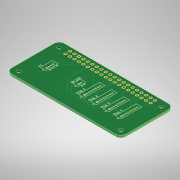
# Autodesk Inventor part: board_main
Saved by Autodesk Inventor 2022.2 (Build 262287010, 287A)
## iProperties
Created: 2025-12-30
Part Number: board_main
Material: Generic
Document SubType Name: Modeling
Designer: dbstj
Density: 1 g/cm^3
Appearance: 매끄러움 - 짙은 산림 녹색
Author: dbstj
Autodesk Inventor part; units mm, degrees
ref_plane "YZ Plane" through (0, 0, 0) normal (1, 0, 0) x (0, 1, 0)
ref_plane "XZ Plane" through (0, 0, 0) normal (0, 1, 0) x (-1, 0, 0)
ref_plane "XY Plane" through (0, 0, 0) normal (0, 0, 1) x (1, 0, 0)
sketch "스케치1" plane through (0, 0, 0) normal (0, 1, 0) x (-1, 0, 0)
  line L0 (-29.5, -15) -> (29.5, -15)
  line L1 (32.5, -12) -> (32.5, 12)
  line L2 (29.5, 15) -> (-29.5, 15)
  line L3 (-32.5, 12) -> (-32.5, -12)
  line L4 (-32.5, -15) -> (32.5, 15) construction
  line L5 (32.5, -15) -> (-32.5, 15) construction
  line L6 (-29, -11.5) -> (29, -11.5)
  line L7 (29, -11.5) -> (29, 11.5)
  line L8 (29, 11.5) -> (-29, 11.5)
  line L9 (-29, 11.5) -> (-29, -11.5)
  line L10 (-29, -11.5) -> (29, 11.5) construction
  line L11 (29, -11.5) -> (-29, 11.5) construction
  circle A0 centre (29, 11.5) radius 1.1
  circle A1 centre (29, -11.5) radius 1.1
  circle A2 centre (-29, -11.5) radius 1.1
  circle A3 centre (-29, 11.5) radius 1.1
  arc A4 (29.5, -15) -> (32.5, -12) centre (29.5, -12) ccw
  arc A5 (-32.5, -12) -> (-29.5, -15) centre (-29.5, -12) ccw
  arc A6 (-29.5, 15) -> (-32.5, 12) centre (-29.5, 12) ccw
  arc A7 (32.5, 12) -> (29.5, 15) centre (29.5, 12) ccw
  point P0 (0, 0)
  point P1 (0, 0)
  point P2 (0, 0)
  dimension "d0" = 65
  dimension "d1" = 30
  dimension "d2" = 58
  dimension "d3" = 23
  dimension "d4" = 2.2
  dimension "d5" = 2.2
  dimension "d6" = 2.2
  dimension "d7" = 2.2
  dimension "d8" = 3
  constraints: 24 end point, 8 centre point, 8 point on circle, 8 point on line, 8 tangent, 5 coincident, 5 midpoint, 4 parallel, 3 equal radius, 2 horizontal, 2 perpendicular
  measures "d0" distance of L5.end L4.end
  measures "d1" distance of L4.end L5.start
  measures "d2" distance of L8.end L7.end
  measures "d3" distance of L7.end L6.end
  measures "d4" diameter of A0
  measures "d5" diameter of A1
  measures "d6" diameter of A2
  measures "d7" diameter of A3
  measures "d8" radius of A4
extrude "돌출1" add sketch "스케치1" along normal blind 1.2 contours A5 L3 A6 L2 A7 L1 A4 L0 | A2 L9 A3 L8 A0 L7 A1 L6
sketch "스케치2" plane through (0, 1.2, 0) normal (0, 1, 0) x (1, 0, 0)
  line L0 (29.5, 15) -> (-29.5, 15) projected
  circle A0 centre (-29, 11.5) radius 1.1 projected
  point P0 (0, 0)
  point P1 (0, 0)
  point P2 (24.13, 12.77)
  point P3 (24.13, 10.23)
  point P4 (21.59, 10.23)
  point P5 (19.05, 12.77)
  point P6 (16.51, 12.77)
  point P7 (13.97, 12.77)
  point P8 (11.43, 12.77)
  point P9 (8.89, 12.77)
  point P10 (6.35, 12.77)
  point P11 (3.81, 12.77)
  point P12 (1.27, 12.77)
  point P13 (-1.27, 12.77)
  point P14 (-3.81, 12.77)
  point P15 (-6.35, 12.77)
  point P16 (-8.89, 12.77)
  point P17 (-11.43, 12.77)
  point P18 (-13.97, 12.77)
  point P19 (-16.51, 12.77)
  point P20 (-19.05, 12.77)
  point P21 (-21.59, 12.77)
  point P22 (19.05, 10.23)
  point P23 (16.51, 10.23)
  point P24 (13.97, 10.23)
  point P25 (11.43, 10.23)
  point P26 (8.89, 10.23)
  point P27 (6.35, 10.23)
  point P28 (3.81, 10.23)
  point P29 (1.27, 10.23)
  point P30 (-1.27, 10.23)
  point P31 (-3.81, 10.23)
  point P32 (-6.35, 10.23)
  point P33 (-8.89, 10.23)
  point P34 (-11.43, 10.23)
  point P35 (-13.97, 10.23)
  point P36 (-16.51, 10.23)
  point P37 (-19.05, 10.23)
  point P38 (-21.59, 10.23)
  point P39 (-24.13, 10.23)
  point P40 (-24.13, 12.77)
  point P41 (21.59, 12.77)
  dimension "d11" = 2.54
  dimension "d12" = 2.54
  dimension "d13" = 2.54
  dimension "d14" = 2.54
  dimension "d15" = 2.54
  dimension "d16" = 2.54
  dimension "d17" = 2.54
  dimension "d18" = 2.54
  dimension "d19" = 2.54
  dimension "d20" = 2.54
  dimension "d21" = 2.54
  dimension "d22" = 2.54
  dimension "d23" = 2.54
  dimension "d24" = 2.54
  dimension "d25" = 2.54
  dimension "d26" = 2.54
  dimension "d27" = 2.54
  dimension "d29" = 2.54
  dimension "d30" = 2.54
  dimension "d31" = 2.54
  dimension "d34" = 27.73
  dimension "d35" = 2.23
  constraints: 38 horizontal alignment, 20 vertical alignment
  measures "d11" distance of point (-21.59, 12.77) point (-19.05, 12.77)
  measures "d12" distance of point (-16.51, 12.77) point (-19.05, 12.77)
  measures "d13" distance of point (-13.97, 12.77) point (-16.51, 12.77)
  measures "d14" distance of point (-11.43, 12.77) point (-13.97, 12.77)
  measures "d15" distance of point (-8.89, 12.77) point (-11.43, 12.77)
  measures "d16" distance of point (-6.35, 12.77) point (-8.89, 12.77)
  measures "d17" distance of point (-3.81, 12.77) point (-6.35, 12.77)
  measures "d18" distance of point (-1.27, 12.77) point (-3.81, 12.77)
  measures "d19" distance of point (1.27, 12.77) point (-1.27, 12.77)
  measures "d20" distance of point (3.81, 12.77) point (1.27, 12.77)
  measures "d21" distance of point (6.35, 12.77) point (3.81, 12.77)
  measures "d22" distance of point (8.89, 12.77) point (6.35, 12.77)
  measures "d23" distance of point (11.43, 12.77) point (8.89, 12.77)
  measures "d24" distance of point (13.97, 12.77) point (11.43, 12.77)
  measures "d25" distance of point (16.51, 12.77) point (13.97, 12.77)
  measures "d26" distance of point (19.05, 12.77) point (16.51, 12.77)
  measures "d27" distance of point (24.13, 12.77) point (24.13, 10.23)
  measures "d29" distance of point (21.59, 12.77) point (19.05, 12.77)
  measures "d30" distance of point (24.13, 12.77) point (21.59, 12.77)
  measures "d31" distance of point (-21.59, 12.77) point (-24.13, 12.77)
  measures "d34" horizontal distance of point (-1.27, 12.77) A0.centre
  measures "d35" distance from line of point (-24.13, 12.77) L0
hole "구멍1" at (24.13, 1.2, -12.77) at (24.13, 1.2, -10.23) at (21.59, 1.2, -10.23) at (19.05, 1.2, -12.77) at (16.51, 1.2, -12.77) at (13.97, 1.2, -12.77) at (11.43, 1.2, -12.77) at (8.89, 1.2, -12.77) at (6.35, 1.2, -12.77) at (3.81, 1.2, -12.77) at (1.27, 1.2, -12.77) at (-1.27, 1.2, -12.77) at (-3.81, 1.2, -12.77) at (-6.35, 1.2, -12.77) at (-8.89, 1.2, -12.77) at (-11.43, 1.2, -12.77) at (-13.97, 1.2, -12.77) at (-16.51, 1.2, -12.77) at (-19.05, 1.2, -12.77) at (-21.59, 1.2, -12.77) at (19.05, 1.2, -10.23) at (16.51, 1.2, -10.23) at (13.97, 1.2, -10.23) at (11.43, 1.2, -10.23) at (8.89, 1.2, -10.23) at (6.35, 1.2, -10.23) at (3.81, 1.2, -10.23) at (1.27, 1.2, -10.23) at (-1.27, 1.2, -10.23) at (-3.81, 1.2, -10.23) at (-6.35, 1.2, -10.23) at (-8.89, 1.2, -10.23) at (-11.43, 1.2, -10.23) at (-13.97, 1.2, -10.23) at (-16.51, 1.2, -10.23) at (-19.05, 1.2, -10.23) at (-21.59, 1.2, -10.23) at (-24.13, 1.2, -10.23) at (-24.13, 1.2, -12.77) at (21.59, 1.2, -12.77) direction (0, -1, 0) diameter 1 end through all
sketch "스케치3" plane through (0, 1.2, 0) normal (0, 1, 0) x (1, 0, 0)
  line L0 (32.5, -12) -> (32.5, 12) projected
  line L1 (29.5, 15) -> (-29.5, 15) projected
  line L2 (-32.5, 12) -> (-32.5, -12) projected
  point P0 (0, 0)
  point P1 (22.5, 4.25)
  point P2 (22.5, 3)
  point P3 (22.5, 1.75)
  point P4 (22.5, 0.5)
  point P5 (22.5, -0.75)
  point P6 (22.5, -2)
  point P7 (22.5, -3.25)
  point P8 (22.5, -4.5)
  point P9 (15.5, -4.5)
  point P10 (15.5, -3.25)
  point P11 (15.5, -2)
  point P12 (15.5, -0.75)
  point P13 (15.5, 0.5)
  point P14 (15.5, 1.75)
  point P15 (15.5, 3)
  point P16 (15.5, 4.25)
  point P17 (8.5, -4.5)
  point P18 (8.5, -3.25)
  point P19 (8.5, -2)
  point P20 (8.5, -0.75)
  point P21 (8.5, 0.5)
  point P22 (8.5, 1.75)
  point P23 (8.5, 3)
  point P24 (8.5, 4.25)
  point P25 (1.5, -4.5)
  point P26 (1.5, -3.25)
  point P27 (1.5, -2)
  point P28 (1.5, -0.75)
  point P29 (1.5, 0.5)
  point P30 (1.5, 1.75)
  point P31 (1.5, 3)
  point P32 (1.5, 4.25)
  point P33 (-5.5, 0.5)
  point P34 (-5.5, -0.75)
  point P35 (-22.5, 1.75)
  point P36 (-22.5, 0.5)
  point P37 (-22.5, -0.75)
  point P38 (-22.5, -2)
  dimension "d43" = 1.25
  dimension "d44" = 1.25
  dimension "d45" = 1.25
  dimension "d46" = 1.25
  dimension "d47" = 1.25
  dimension "d48" = 1.25
  dimension "d49" = 1.25
  dimension "d50" = 10
  dimension "d54" = 7
  dimension "d59" = 1.25
  dimension "d60" = 1.25
  dimension "d61" = 1.25
  dimension "d62" = 1.25
  dimension "d64" = 10
  dimension "d65" = 7
  dimension "d73" = 19.5
  dimension "d74" = 15.75
  dimension "d75" = 17
  constraints: 11 vertical alignment, 2 horizontal alignment, 1 horizontal, 24 other
  measures "d43" distance of point (22.5, 3) point (22.5, 4.25)
  measures "d44" distance of point (22.5, 1.75) point (22.5, 3)
  measures "d45" distance of point (22.5, 0.5) point (22.5, 1.75)
  measures "d46" distance of point (22.5, -0.75) point (22.5, 0.5)
  measures "d47" distance of point (22.5, -0.75) point (22.5, -2)
  measures "d48" distance of point (22.5, -2) point (22.5, -3.25)
  measures "d49" distance of point (22.5, -3.25) point (22.5, -4.5)
  measures "d50" distance from line of L0 point (22.5, 4.25)
  measures "d54" distance of point (22.5, -4.5) point (15.5, -4.5)
  measures "d59" distance of point (-22.5, 0.5) point (-22.5, 1.75)
  measures "d60" distance of point (-22.5, -0.75) point (-22.5, 0.5)
  measures "d61" distance of point (-22.5, -2) point (-22.5, -0.75)
  measures "d62" distance of point (-5.5, -0.75) point (-5.5, 0.5)
  measures "d64" distance from line of L2 point (-22.5, 1.75)
  measures "d65" horizontal distance of point (1.5, 4.25) point (-5.5, 0.5)
  measures "d73" distance from line of L1 point (22.5, -4.5)
  measures "d74" distance from line of L1 point (-5.5, -0.75)
  measures "d75" distance from line of L1 point (-22.5, -2)
hole "구멍2" at (22.5, 1.2, -4.25) at (22.5, 1.2, -3) at (22.5, 1.2, -1.75) at (22.5, 1.2, -0.5) at (22.5, 1.2, 0.75) at (22.5, 1.2, 2) at (22.5, 1.2, 3.25) at (22.5, 1.2, 4.5) at (15.5, 1.2, 4.5) at (15.5, 1.2, 3.25) at (15.5, 1.2, 2) at (15.5, 1.2, 0.75) at (15.5, 1.2, -0.5) at (15.5, 1.2, -1.75) at (15.5, 1.2, -3) at (15.5, 1.2, -4.25) at (8.5, 1.2, 4.5) at (8.5, 1.2, 3.25) at (8.5, 1.2, 2) at (8.5, 1.2, 0.75) at (8.5, 1.2, -0.5) at (8.5, 1.2, -1.75) at (8.5, 1.2, -3) at (8.5, 1.2, -4.25) at (1.5, 1.2, 4.5) at (1.5, 1.2, 3.25) at (1.5, 1.2, 2) at (1.5, 1.2, 0.75) at (1.5, 1.2, -0.5) at (1.5, 1.2, -1.75) at (1.5, 1.2, -3) at (1.5, 1.2, -4.25) at (-5.5, 1.2, -0.5) at (-5.5, 1.2, 0.75) at (-22.5, 1.2, -1.75) at (-22.5, 1.2, -0.5) at (-22.5, 1.2, 0.75) at (-22.5, 1.2, 2) direction (0, -1, 0) diameter 0.6 end through all
sketch "스케치4" plane through (0, 1.2, 0) normal (0, 1, 0) x (1, 0, 0)
  circle A0 centre (-22.5, -0.75) radius 0.3 projected
  circle A1 centre (-22.5, 1.75) radius 0.3 projected
  circle A2 centre (-5.5, 0.5) radius 0.3 projected
  circle A3 centre (1.5, 3) radius 0.3 projected
  circle A4 centre (1.5, 0.5) radius 0.3 projected
  circle A5 centre (1.5, -2) radius 0.3 projected
  circle A6 centre (1.5, -4.5) radius 0.3 projected
  circle A7 centre (8.5, 3) radius 0.3 projected
  circle A8 centre (8.5, 0.5) radius 0.3 projected
  circle A9 centre (8.5, -2) radius 0.3 projected
  circle A10 centre (8.5, -4.5) radius 0.3 projected
  circle A11 centre (15.5, 3) radius 0.3 projected
  circle A12 centre (15.5, 0.5) radius 0.3 projected
  circle A13 centre (15.5, -2) radius 0.3 projected
  circle A14 centre (15.5, -4.5) radius 0.3 projected
  circle A15 centre (22.5, -3.25) radius 0.3 projected
  circle A16 centre (22.5, -0.75) radius 0.3 projected
  circle A17 centre (22.5, 1.75) radius 0.3 projected
  circle A18 centre (22.5, 4.25) radius 0.3 projected
  circle A19 centre (22.5, 3) radius 0.3 projected
  circle A20 centre (22.5, 0.5) radius 0.3 projected
  circle A21 centre (22.5, -2) radius 0.3 projected
  circle A22 centre (22.5, -4.5) radius 0.3 projected
  circle A23 centre (15.5, -3.25) radius 0.3 projected
  circle A24 centre (15.5, -0.75) radius 0.3 projected
  circle A25 centre (15.5, 1.75) radius 0.3 projected
  circle A26 centre (15.5, 4.25) radius 0.3 projected
  circle A27 centre (8.5, -3.25) radius 0.3 projected
  circle A28 centre (8.5, -0.75) radius 0.3 projected
  circle A29 centre (8.5, 1.75) radius 0.3 projected
  circle A30 centre (8.5, 4.25) radius 0.3 projected
  circle A31 centre (1.5, -3.25) radius 0.3 projected
  circle A32 centre (1.5, -0.75) radius 0.3 projected
  circle A33 centre (1.5, 1.75) radius 0.3 projected
  circle A34 centre (1.5, 4.25) radius 0.3 projected
  circle A35 centre (-5.5, -0.75) radius 0.3 projected
  circle A36 centre (-22.5, 0.5) radius 0.3 projected
  circle A37 centre (-22.5, -2) radius 0.3 projected
  circle A38 centre (-24.13, 12.77) radius 0.5 projected
  circle A39 centre (-21.59, 10.23) radius 0.5 projected
  circle A40 centre (-16.51, 10.23) radius 0.5 projected
  circle A41 centre (-11.43, 10.23) radius 0.5 projected
  circle A42 centre (-6.35, 10.23) radius 0.5 projected
  circle A43 centre (-1.27, 10.23) radius 0.5 projected
  circle A44 centre (3.81, 10.23) radius 0.5 projected
  circle A45 centre (8.89, 10.23) radius 0.5 projected
  circle A46 centre (13.97, 10.23) radius 0.5 projected
  circle A47 centre (19.05, 10.23) radius 0.5 projected
  circle A48 centre (-19.05, 12.77) radius 0.5 projected
  circle A49 centre (-13.97, 12.77) radius 0.5 projected
  circle A50 centre (-8.89, 12.77) radius 0.5 projected
  circle A51 centre (-3.81, 12.77) radius 0.5 projected
  circle A52 centre (1.27, 12.77) radius 0.5 projected
  circle A53 centre (6.35, 12.77) radius 0.5 projected
  circle A54 centre (11.43, 12.77) radius 0.5 projected
  circle A55 centre (16.51, 12.77) radius 0.5 projected
  circle A56 centre (21.59, 10.23) radius 0.5 projected
  circle A57 centre (24.13, 12.77) radius 0.5 projected
  circle A58 centre (24.13, 10.23) radius 0.5 projected
  circle A59 centre (19.05, 12.77) radius 0.5 projected
  circle A60 centre (13.97, 12.77) radius 0.5 projected
  circle A61 centre (8.89, 12.77) radius 0.5 projected
  circle A62 centre (3.81, 12.77) radius 0.5 projected
  circle A63 centre (-1.27, 12.77) radius 0.5 projected
  circle A64 centre (-6.35, 12.77) radius 0.5 projected
  circle A65 centre (-11.43, 12.77) radius 0.5 projected
  circle A66 centre (-16.51, 12.77) radius 0.5 projected
  circle A67 centre (-21.59, 12.77) radius 0.5 projected
  circle A68 centre (16.51, 10.23) radius 0.5 projected
  circle A69 centre (11.43, 10.23) radius 0.5 projected
  circle A70 centre (6.35, 10.23) radius 0.5 projected
  circle A71 centre (1.27, 10.23) radius 0.5 projected
  circle A72 centre (-3.81, 10.23) radius 0.5 projected
  circle A73 centre (-8.89, 10.23) radius 0.5 projected
  circle A74 centre (-13.97, 10.23) radius 0.5 projected
  circle A75 centre (-19.05, 10.23) radius 0.5 projected
  circle A76 centre (-24.13, 10.23) radius 0.5 projected
  circle A77 centre (21.59, 12.77) radius 0.5 projected
  arc A78 (-29.5, 15) -> (-32.5, 12) centre (-29.5, 12) ccw projected
  line L0 (-32.5, 12) -> (-32.5, -12) projected
  arc A79 (-32.5, -12) -> (-29.5, -15) centre (-29.5, -12) ccw projected
  line L1 (-29.5, -15) -> (29.5, -15) projected
  arc A80 (29.5, -15) -> (32.5, -12) centre (29.5, -12) ccw projected
  line L2 (32.5, -12) -> (32.5, 12) projected
  arc A81 (32.5, 12) -> (29.5, 15) centre (29.5, 12) ccw projected
  line L3 (29.5, 15) -> (-29.5, 15) projected
  circle A82 centre (29, -11.5) radius 1.1 projected
  circle A83 centre (29, 11.5) radius 1.1 projected
  circle A84 centre (-29, 11.5) radius 1.1 projected
  circle A85 centre (-29, -11.5) radius 1.1 projected
  line L4 (-32.7525, -15.271) -> (-32.7525, 15.4111) construction
  line L5 (-32.7525, 15.4111) -> (32.7686, 15.4111) construction
  line L6 (32.7686, 15.4111) -> (32.7686, -15.271) construction
  line L7 (32.7686, -15.271) -> (-32.7525, -15.271) construction
  point P0 (0, 0)
  constraints: 1 parallel, 2 other
decal "전사1"
sketch "스케치5" plane through (0, 0, 0) normal (0, -1, 0) x (1, 0, 0)
  circle A0 centre (-22.5, 0.75) radius 0.3 projected
  circle A1 centre (-22.5, -1.75) radius 0.3 projected
  circle A2 centre (-5.5, -0.5) radius 0.3 projected
  circle A3 centre (1.5, -3) radius 0.3 projected
  circle A4 centre (1.5, -0.5) radius 0.3 projected
  circle A5 centre (1.5, 2) radius 0.3 projected
  circle A6 centre (1.5, 4.5) radius 0.3 projected
  circle A7 centre (8.5, -3) radius 0.3 projected
  circle A8 centre (8.5, -0.5) radius 0.3 projected
  circle A9 centre (8.5, 2) radius 0.3 projected
  circle A10 centre (8.5, 4.5) radius 0.3 projected
  circle A11 centre (15.5, -3) radius 0.3 projected
  circle A12 centre (15.5, -0.5) radius 0.3 projected
  circle A13 centre (15.5, 2) radius 0.3 projected
  circle A14 centre (15.5, 4.5) radius 0.3 projected
  circle A15 centre (22.5, 3.25) radius 0.3 projected
  circle A16 centre (22.5, 0.75) radius 0.3 projected
  circle A17 centre (22.5, -1.75) radius 0.3 projected
  circle A18 centre (22.5, -4.25) radius 0.3 projected
  circle A19 centre (22.5, -3) radius 0.3 projected
  circle A20 centre (22.5, -0.5) radius 0.3 projected
  circle A21 centre (22.5, 2) radius 0.3 projected
  circle A22 centre (22.5, 4.5) radius 0.3 projected
  circle A23 centre (15.5, 3.25) radius 0.3 projected
  circle A24 centre (15.5, 0.75) radius 0.3 projected
  circle A25 centre (15.5, -1.75) radius 0.3 projected
  circle A26 centre (15.5, -4.25) radius 0.3 projected
  circle A27 centre (8.5, 3.25) radius 0.3 projected
  circle A28 centre (8.5, 0.75) radius 0.3 projected
  circle A29 centre (8.5, -1.75) radius 0.3 projected
  circle A30 centre (8.5, -4.25) radius 0.3 projected
  circle A31 centre (1.5, 3.25) radius 0.3 projected
  circle A32 centre (1.5, 0.75) radius 0.3 projected
  circle A33 centre (1.5, -1.75) radius 0.3 projected
  circle A34 centre (1.5, -4.25) radius 0.3 projected
  circle A35 centre (-5.5, 0.75) radius 0.3 projected
  circle A36 centre (-22.5, -0.5) radius 0.3 projected
  circle A37 centre (-22.5, 2) radius 0.3 projected
  circle A38 centre (-24.13, -12.77) radius 0.5 projected
  circle A39 centre (-21.59, -10.23) radius 0.5 projected
  circle A40 centre (-16.51, -10.23) radius 0.5 projected
  circle A41 centre (-11.43, -10.23) radius 0.5 projected
  circle A42 centre (-6.35, -10.23) radius 0.5 projected
  circle A43 centre (-1.27, -10.23) radius 0.5 projected
  circle A44 centre (3.81, -10.23) radius 0.5 projected
  circle A45 centre (8.89, -10.23) radius 0.5 projected
  circle A46 centre (13.97, -10.23) radius 0.5 projected
  circle A47 centre (19.05, -10.23) radius 0.5 projected
  circle A48 centre (-19.05, -12.77) radius 0.5 projected
  circle A49 centre (-13.97, -12.77) radius 0.5 projected
  circle A50 centre (-8.89, -12.77) radius 0.5 projected
  circle A51 centre (-3.81, -12.77) radius 0.5 projected
  circle A52 centre (1.27, -12.77) radius 0.5 projected
  circle A53 centre (6.35, -12.77) radius 0.5 projected
  circle A54 centre (11.43, -12.77) radius 0.5 projected
  circle A55 centre (16.51, -12.77) radius 0.5 projected
  circle A56 centre (21.59, -10.23) radius 0.5 projected
  circle A57 centre (24.13, -12.77) radius 0.5 projected
  circle A58 centre (24.13, -10.23) radius 0.5 projected
  circle A59 centre (19.05, -12.77) radius 0.5 projected
  circle A60 centre (13.97, -12.77) radius 0.5 projected
  circle A61 centre (8.89, -12.77) radius 0.5 projected
  circle A62 centre (3.81, -12.77) radius 0.5 projected
  circle A63 centre (-1.27, -12.77) radius 0.5 projected
  circle A64 centre (-6.35, -12.77) radius 0.5 projected
  circle A65 centre (-11.43, -12.77) radius 0.5 projected
  circle A66 centre (-16.51, -12.77) radius 0.5 projected
  circle A67 centre (-21.59, -12.77) radius 0.5 projected
  circle A68 centre (16.51, -10.23) radius 0.5 projected
  circle A69 centre (11.43, -10.23) radius 0.5 projected
  circle A70 centre (6.35, -10.23) radius 0.5 projected
  circle A71 centre (1.27, -10.23) radius 0.5 projected
  circle A72 centre (-3.81, -10.23) radius 0.5 projected
  circle A73 centre (-8.89, -10.23) radius 0.5 projected
  circle A74 centre (-13.97, -10.23) radius 0.5 projected
  circle A75 centre (-19.05, -10.23) radius 0.5 projected
  circle A76 centre (-24.13, -10.23) radius 0.5 projected
  circle A77 centre (21.59, -12.77) radius 0.5 projected
  arc A78 (-32.5, -12) -> (-29.5, -15) centre (-29.5, -12) ccw projected
  line L0 (29.5, -15) -> (-29.5, -15) projected
  arc A79 (29.5, -15) -> (32.5, -12) centre (29.5, -12) ccw projected
  line L1 (32.5, 12) -> (32.5, -12) projected
  arc A80 (32.5, 12) -> (29.5, 15) centre (29.5, 12) ccw projected
  line L2 (-29.5, 15) -> (29.5, 15) projected
  arc A81 (-29.5, 15) -> (-32.5, 12) centre (-29.5, 12) ccw projected
  line L3 (-32.5, -12) -> (-32.5, 12) projected
  circle A82 centre (29, 11.5) radius 1.1 projected
  circle A83 centre (29, -11.5) radius 1.1 projected
  circle A84 centre (-29, -11.5) radius 1.1 projected
  circle A85 centre (-29, 11.5) radius 1.1 projected
  line L4 (-32.8409, -15.4192) -> (-32.8409, 15.3937) construction
  line L5 (-32.8409, 15.3937) -> (32.8757, 15.3937) construction
  line L6 (32.8757, 15.3937) -> (32.8757, -15.4192) construction
  line L7 (32.8757, -15.4192) -> (-32.8409, -15.4192) construction
  line L8 (-29.5, 15) -> (29.5, 15) projected
  point P0 (0, 0)
  constraints: 1 parallel, 2 other
decal "전사2"
equation "\"d4\" = d5"
equation "\"d6\" = d5"
equation "\"d7\" = d5"
equation "\"d11\" = d33"
equation "\"d12\" = d33"
equation "\"d13\" = d33"
equation "\"d14\" = d33"
equation "\"d15\" = d33"
equation "\"d16\" = d33"
equation "\"d17\" = d33"
equation "\"d18\" = d33"
equation "\"d19\" = d33"
equation "\"d20\" = d33"
equation "\"d21\" = d33"
equation "\"d22\" = d33"
equation "\"d23\" = d33"
equation "\"d24\" = d33"
equation "\"d25\" = d33"
equation "\"d26\" = d33"
equation "\"d29\" = d26"
equation "\"d30\" = d26"
equation "\"d31\" = d11"
equation "\"d44\" = d43"
equation "\"d45\" = d43"
equation "\"d46\" = d43"
equation "\"d47\" = d43"
equation "\"d48\" = d43"
equation "\"d49\" = d43"
equation "\"d60\" = d59"
equation "\"d61\" = d59"
equation "\"d33\" = 2.54"
